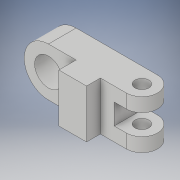
# Autodesk Inventor part: Součást15
Saved by Autodesk Inventor 2019 (Build 230136000, 136)
## iProperties
Created: 2019-12-16
Part Number: Součást15
Material: Všeobecné
Document SubType Name: Modeling
Designer: hynek
Density: 1 g/cm^3
Appearance: Výchozí
Author: hynek
Autodesk Inventor part; units mm, degrees
ref_plane "YZ Plane" through (0, 0, 0) normal (1, 0, 0) x (0, 1, 0)
ref_plane "XZ Plane" through (0, 0, 0) normal (0, 1, 0) x (-1, 0, 0)
ref_plane "XY Plane" through (0, 0, 0) normal (0, 0, 1) x (1, 0, 0)
sketch "Náčrt1" plane through (0, 0, 0) normal (0, 0, 1) x (1, 0, 0)
  circle A0 centre (0, 0) radius 4
  arc A1 (0, 7) -> (0, -7) centre (0, 0) ccw
  line L0 (0, -9.8) -> (0, 9.8) construction
  line L1 (-14, 0) -> (35, 0) construction
  line L2 (0, -7) -> (28, -7)
  line L3 (28, -7) -> (28, -3)
  line L4 (28, -3) -> (20, -3)
  line L5 (20, -3) -> (20, 3)
  line L6 (20, 3) -> (28, 3)
  line L7 (28, 3) -> (28, 7)
  line L8 (28, 7) -> (0, 7)
  dimension "d0" = 8
  dimension "d1" = 14
  dimension "d2" = 4
  dimension "d3" = 4
  dimension "d4" = 6
  dimension "d5" = 8
  dimension "d6" = 28
  constraints: 14 end point, 5 perpendicular, 3 point on line, 2 centre point, 2 coincident, 2 point on circle, 2 tangent
  measures "d0" diameter of A0
  measures "d1" diameter of A1
  measures "d2" distance between parallel lines of L2 L4
  measures "d3" distance between parallel lines of L6 L8
  measures "d4" distance between parallel lines of L6 L4
  measures "d5" distance between parallel lines of L3 L5
  measures "d6" distance between parallel lines of L0 L3
extrude "Vysunutí1" add sketch "Náčrt1" along normal blind 8
sketch "Náčrt2" plane through (0, 0, 8) normal (0, 0, 1) x (1, 0, 0)
  line L0 (-14, 0) -> (35, 0) construction
  line L1 (0, -9.8) -> (0, 9.8) construction
  line L2 (8, 7) -> (16, 7)
  line L3 (16, 7) -> (16, -7)
  line L4 (16, -7) -> (8, -7)
  line L5 (8, -7) -> (8, 7)
  point P0 (0, 0)
  dimension "d10" = 8
  dimension "d11" = 8
  dimension "d12" = 7
  dimension "d13" = 7
  constraints: 8 end point, 2 parallel, 1 horizontal, 1 perpendicular
  measures "d10" distance between parallel lines of L1 L5
  measures "d11" distance between parallel lines of L5 L3
  measures "d12" distance between parallel lines of L0 L4
  measures "d13" distance between parallel lines of L0 L2
extrude "Vysunutí2" add sketch "Náčrt2" along normal blind 5
sketch "Náčrt5" plane through (0, 0, 8) normal (0, 0, 1) x (1, 0, 0)
  line L0 (16, 7) -> (16, -7) projected
  line L1 (16, -7) -> (28, -7) projected
  line L2 (28, -7) -> (28, -3) projected
  line L3 (28, -3) -> (20, -3) projected
  line L4 (20, -3) -> (20, 3) projected
  line L5 (20, 3) -> (28, 3) projected
  line L6 (28, 3) -> (28, 7) projected
  line L7 (28, 7) -> (16, 7) projected
  point P0 (0, 0)
extrude "Vysunutí4" add sketch "Náčrt5" along normal blind 1
sketch "Náčrt6" plane through (0, -7, 0) normal (0, -1, 0) x (1, 0, 0)
  point P0 (0, 0)
fillet "Zaoblení2" radius 4.5 4 edges at (28, -5, 9) (28, -5, 0) (28, 5, 0) (28, 5, 9)
sketch "Náčrt7" plane through (0, -7, 0) normal (0, -1, 0) x (1, 0, 0)
  arc A0 (23.5, 0) -> (23.5, 9) centre (23.5, 4.5) ccw construction
  circle A1 centre (23.5, 4.5) radius 2
  point P0 (0, 0)
  dimension "d22" = 4
  constraints: 1 centre point, 1 coincident
  measures "d22" diameter of A1
extrude "Vysunutí5" cut sketch "Náčrt7" against normal through all
